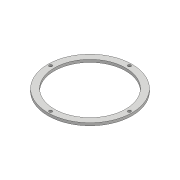
# Autodesk Inventor part: arm_0_bottom_top_lock
Saved by Autodesk Inventor 2018 (Build 220112000, 112)
## iProperties
Created: 2017-12-04
Part Number: arm_0_bottom_top_lock
Material: Generic
Document SubType Name: Modeling
Designer: Bardo91
Density: 1 g/cm^3
Appearance: Default
Mass: 5.88047 g
Surface Area: 57.0631 cm^2
Volume: 5.88047 cm^3
Author: Bardo91
Autodesk Inventor part; units mm, degrees
ref_plane "YZ Plane" through (0, 0, 0) normal (1, 0, 0) x (0, 1, 0)
ref_plane "XZ Plane" through (0, 0, 0) normal (0, 1, 0) x (-1, 0, 0)
ref_plane "XY Plane" through (0, 0, 0) normal (0, 0, 1) x (1, 0, 0)
sketch "Sketch1" plane through (0, 0, 0) normal (0, 0, 1) x (1, 0, 0)
  circle A0 centre (0, 0) radius 48
  circle A1 centre (0, 0) radius 40.75
  line L0 (0, 0) -> (0, 45)
  circle A2 centre (0, 45) radius 1.75
  circle A3 centre (-45, 0) radius 1.75
  circle A4 centre (0, -45) radius 1.75
  circle A5 centre (45, 0) radius 1.75
  dimension "d0" = 96
  dimension "d1" = 81.5
  dimension "d2" = 45
  dimension "d3" = 3.5
  dimension "d6" = 360
  constraints: 6 centre point, 5 coincident, 2 end point, 1 vertical, 11 other
  measures "d0" diameter of A0
  measures "d1" diameter of A1
  measures "d2" distance of L0.start L0.end
  measures "d3" diameter of A2
extrude "Extrusion1" add sketch "Sketch1" along normal blind 3
body "Solid1"
